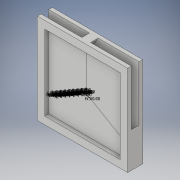
# Autodesk Inventor part: end door
Saved by Autodesk Inventor 2017 (Build 210142000, 142)
## iProperties
Created: 2018-03-09
Part Number: end door
Material: Generic
Document SubType Name: Modeling
Designer: Braxton
Density: 1 g/cm^3
Appearance: Default
Author: Braxton
Autodesk Inventor part; units mm, degrees
ref_plane "YZ Plane" through (0, 0, 0) normal (1, 0, 0) x (0, 1, 0)
ref_plane "XZ Plane" through (0, 0, 0) normal (0, 1, 0) x (-1, 0, 0)
ref_plane "XY Plane" through (0, 0, 0) normal (0, 0, 1) x (1, 0, 0)
sketch "Sketch1" plane through (0, 0, 0) normal (0, 0, 1) x (1, 0, 0)
  line L0 (0, 0) -> (2540, 0)
  line L1 (2540, 0) -> (2540, 2540)
  line L2 (2540, 2540) -> (0, 2540)
  line L3 (0, 2540) -> (0, 0)
  line L4 (-254, 2794) -> (2794, 2794)
  line L5 (2794, 2794) -> (2794, -254)
  line L6 (2794, -254) -> (-254, -254)
  line L7 (-254, -254) -> (-254, 2794)
  dimension "d0" = 2540
  dimension "d1" = 2540
  dimension "d3" = 254
  dimension "d4" = 254
  dimension "d5" = 254
  dimension "d6" = 254
  constraints: 16 end point, 4 perpendicular, 2 horizontal, 2 parallel
  measures "d0" distance of L0.start L0.end
  measures "d1" distance of L0.end L1.end
  measures "d3" distance between parallel lines of L2 L4
  measures "d4" distance between parallel lines of L3 L7
  measures "d5" distance between parallel lines of L5 L1
  measures "d6" distance between parallel lines of L6 L0
extrude "frame" add sketch "Sketch1" along normal mid plane 508
ref_plane "Work Plane3" through (0, 0, 0) normal (0, 0, 1) x (1, 0, 0)
sketch "Sketch8" plane through (0, 0, 0) normal (0, 0, 1) x (1, 0, 0)
  line L0 (2540, 0) -> (0, 0) projected
  line L1 (0, 0) -> (0, -254)
  line L2 (-254, -254) -> (2794, -254) projected
  line L3 (0, -254) -> (2540, -254)
  line L4 (2540, 2540) -> (2540, 0) projected
  line L5 (2540, -254) -> (2540, 0)
  line L6 (2540, 0) -> (0, 0)
  constraints: 8 end point, 3 perpendicular, 1 point on line, 1 vertical
extrude "door slot bottom" cut sketch "Sketch8" along normal mid plane 254
sketch "Sketch5" plane through (0, 0, 0) normal (0, 0, 1) x (1, 0, 0)
  line L0 (0, 0) -> (0, 2540) projected
  line L1 (2540, 0) -> (2540, 2540) projected
  line L2 (1270, 1143) -> (1270, 970.0002) construction
  line L3 (0, 0) -> (2540, 0) projected
  line L4 (0, 498.8101) -> (0, 0)
  line L5 (0, 0) -> (2540, 0)
  line L6 (2540, 0) -> (2540, 498.8101)
  line L7 (1270, 1232.045) -> (0, 498.8101)
  line L8 (1270, 1232.045) -> (2540, 498.8101)
  line L9 (0, 498.8101) -> (0, 2540)
  line L10 (0, 2540) -> (1270, 2540)
  line L11 (2540, 2540) -> (0, 2540) projected
  line L12 (1270, 2540) -> (1270, 1232.045)
  line L13 (1270, 2540) -> (2540, 2540)
  line L14 (2540, 2540) -> (2540, 498.8101)
  dimension "d247" = 60
  dimension "d248" = 60
  constraints: 22 end point, 3 perpendicular, 2 collinear, 2 point on line, 2 vertical, 1 horizontal, 1 midpoint
  measures "d247" angle of L7 L2
  measures "d248" angle of L8 L2
extrude "doors sketch" add sketch "Sketch5" along normal mid plane 254 separate body contours L0 L7 L8 L1 L3
extrude "top left door" add sketch "Sketch5" along normal mid plane 254 separate body contours L0 L10 L12 L7
extrude "top right door" add sketch "Sketch5" along normal mid plane 254 separate body contours L12 L11 L1 L8
sketch "Sketch7" plane through (0, 0, 0) normal (0, 0, 1) x (1, 0, 0)
  line L0 (106.265, 560.1623) -> (-264.3091, 1202.0154) construction
  line L1 (0, 498.8101) -> (-254, 938.751)
  line L2 (1270, 1232.045) -> (2540, 498.8101) projected
  line L3 (1270, 1232.045) -> (1270, 2794) construction
  line L4 (-254, 2794) -> (2794, 2794) projected
  line L5 (2540, 2540) -> (0, 2540) projected
  line L6 (1270, 2540) -> (1123.353, 2794)
  line L7 (-254, -254) -> (-254, 2794) projected
  line L8 (1123.353, 2794) -> (-254, 2794)
  line L9 (-254, 2794) -> (-254, 938.751)
  line L10 (0, 2540) -> (1270, 2540)
  line L11 (0, 498.8101) -> (1270, 1232.045) projected
  line L12 (0, 2540) -> (0, 498.8101)
  line L13 (2540, 498.8101) -> (2794, 938.751)
  line L14 (1270, 2540) -> (1416.647, 2794)
  line L15 (1416.647, 2794) -> (2794, 2794)
  line L16 (2794, 2794) -> (2794, 938.751)
  line L17 (2540, 2540) -> (1270, 2540)
  line L18 (2540, 2540) -> (2540, 498.8101)
  constraints: 28 end point, 3 point on line, 2 midpoint, 2 parallel, 2 symmetric about line, 1 horizontal, 1 perpendicular, 1 vertical
extrude "top left and right slots" cut sketch "Sketch7" along normal mid plane 254 contours L1 L7 L4 L6 L5 L12 | L18 L5 L14 L4 L16 L13 bodies 1
sketch "Sketch6" plane through (0, 0, 0) normal (0, 0, 1) x (1, 0, 0)
  line L0 (1270, 1324.5674) -> (1270, 1217.3803) construction
  line L1 (35.592, 519.3592) -> (22.892, 541.3562) construction
  line L2 (11.8934, 535.0062) -> (33.8905, 547.7062)
  line L3 (11.8934, 535.0062) -> (0, 498.8101)
  line L4 (119.4759, 538.4602) -> (106.7759, 560.4572) construction
  line L5 (108.4774, 532.1102) -> (130.4744, 544.8102)
  line L6 (71.1839, 539.9082) -> (108.4774, 532.1102)
  line L7 (33.8905, 547.7062) -> (71.1839, 539.9082)
  line L8 (130.4744, 544.8102) -> (142.3679, 581.0063)
  line L9 (1270, 1232.045) -> (2540, 498.8101) projected
  line L10 (0, 498.8101) -> (1270, 1232.045) projected
  line L11 (272.8423, 627.0063) -> (284.7357, 663.2024)
  line L12 (250.8452, 614.3063) -> (272.8423, 627.0063)
  line L13 (213.5518, 622.1043) -> (250.8452, 614.3063)
  line L14 (176.2584, 629.9023) -> (213.5518, 622.1043)
  line L15 (177.9598, 601.5553) -> (165.2598, 623.5523) construction
  line L16 (154.2613, 617.2023) -> (176.2584, 629.9023)
  line L17 (154.2613, 617.2023) -> (142.3679, 581.0063)
  line L18 (261.8438, 620.6563) -> (249.1438, 642.6534) construction
  line L19 (415.2102, 709.2024) -> (427.1036, 745.3985)
  line L20 (393.2131, 696.5024) -> (415.2102, 709.2024)
  line L21 (355.9197, 704.3004) -> (393.2131, 696.5024)
  line L22 (318.6262, 712.0985) -> (355.9197, 704.3004)
  line L23 (320.3277, 683.7514) -> (307.6277, 705.7485) construction
  line L24 (296.6292, 699.3985) -> (318.6262, 712.0985)
  line L25 (296.6292, 699.3985) -> (284.7357, 663.2024)
  line L26 (404.2116, 702.8524) -> (391.5116, 724.8495) construction
  line L27 (557.578, 791.3986) -> (569.4715, 827.5946)
  line L28 (535.581, 778.6986) -> (557.578, 791.3986)
  line L29 (498.2875, 786.4966) -> (535.581, 778.6986)
  line L30 (460.9941, 794.2946) -> (498.2875, 786.4966)
  line L31 (462.6956, 765.9475) -> (449.9956, 787.9446) construction
  line L32 (438.997, 781.5946) -> (460.9941, 794.2946)
  line L33 (438.997, 781.5946) -> (427.1036, 745.3985)
  line L34 (546.5795, 785.0486) -> (533.8795, 807.0456) construction
  line L35 (699.9459, 873.5947) -> (711.8393, 909.7908)
  line L36 (677.9488, 860.8947) -> (699.9459, 873.5947)
  line L37 (640.6554, 868.6927) -> (677.9488, 860.8947)
  line L38 (603.362, 876.4907) -> (640.6554, 868.6927)
  line L39 (605.0634, 848.1437) -> (592.3634, 870.1407) construction
  line L40 (581.3649, 863.7907) -> (603.362, 876.4907)
  line L41 (581.3649, 863.7907) -> (569.4715, 827.5946)
  line L42 (688.9474, 867.2447) -> (676.2474, 889.2417) construction
  line L43 (842.3138, 955.7908) -> (854.2072, 991.9869)
  line L44 (820.3167, 943.0908) -> (842.3138, 955.7908)
  line L45 (783.0233, 950.8888) -> (820.3167, 943.0908)
  line L46 (745.7298, 958.6868) -> (783.0233, 950.8888)
  line L47 (747.4313, 930.3398) -> (734.7313, 952.3368) construction
  line L48 (723.7328, 945.9868) -> (745.7298, 958.6868)
  line L49 (723.7328, 945.9868) -> (711.8393, 909.7908)
  line L50 (831.3152, 949.4408) -> (818.6152, 971.4379) construction
  line L51 (984.6816, 1037.9869) -> (996.5751, 1074.183)
  line L52 (962.6846, 1025.2869) -> (984.6816, 1037.9869)
  line L53 (925.3911, 1033.085) -> (962.6846, 1025.2869)
  line L54 (888.0977, 1040.883) -> (925.3911, 1033.085)
  line L55 (889.7992, 1012.5359) -> (877.0992, 1034.533) construction
  line L56 (866.1006, 1028.183) -> (888.0977, 1040.883)
  line L57 (866.1006, 1028.183) -> (854.2072, 991.9869)
  line L58 (973.6831, 1031.6369) -> (960.9831, 1053.634) construction
  line L59 (1127.0495, 1120.1831) -> (1138.9429, 1156.3791)
  line L60 (1105.0525, 1107.4831) -> (1127.0495, 1120.1831)
  line L61 (1067.759, 1115.2811) -> (1105.0525, 1107.4831)
  line L62 (1030.4656, 1123.0791) -> (1067.759, 1115.2811)
  line L63 (1032.167, 1094.732) -> (1019.467, 1116.7291) construction
  line L64 (1008.4685, 1110.3791) -> (1030.4656, 1123.0791)
  line L65 (1008.4685, 1110.3791) -> (996.5751, 1074.183)
  line L66 (1116.051, 1113.8331) -> (1103.351, 1135.8301) construction
  line L67 (1172.8334, 1205.2752) -> (1210.1269, 1197.4772)
  line L68 (1174.5349, 1176.9282) -> (1161.8349, 1198.9252) construction
  line L69 (1150.8364, 1192.5752) -> (1172.8334, 1205.2752)
  line L70 (1150.8364, 1192.5752) -> (1138.9429, 1156.3791)
  line L71 (0, 498.8101) -> (71.1839, 539.9082)
  line L72 (71.1839, 539.9082) -> (142.3679, 581.0063)
  line L73 (142.3679, 581.0063) -> (213.5518, 622.1043)
  line L74 (213.5518, 622.1043) -> (284.7357, 663.2024)
  line L75 (284.7357, 663.2024) -> (355.9197, 704.3004)
  line L76 (355.9197, 704.3004) -> (427.1036, 745.3985)
  line L77 (427.1036, 745.3985) -> (498.2875, 786.4966)
  line L78 (498.2875, 786.4966) -> (569.4715, 827.5946)
  line L79 (569.4715, 827.5946) -> (640.6554, 868.6927)
  line L80 (640.6554, 868.6927) -> (711.8393, 909.7908)
  line L81 (711.8393, 909.7908) -> (783.0233, 950.8888)
  line L82 (783.0233, 950.8888) -> (854.2072, 991.9869)
  line L83 (854.2072, 991.9869) -> (925.3911, 1033.085)
  line L84 (925.3911, 1033.085) -> (996.5751, 1074.183)
  line L85 (996.5751, 1074.183) -> (1067.759, 1115.2811)
  line L86 (1067.759, 1115.2811) -> (1138.9429, 1156.3791)
  line L87 (1138.9429, 1156.3791) -> (1210.1269, 1197.4772)
  line L88 (2409.5256, 544.8102) -> (2397.6321, 581.0063)
  line L89 (2431.5226, 532.1102) -> (2409.5256, 544.8102)
  line L90 (2468.8161, 539.9082) -> (2431.5226, 532.1102)
  line L91 (2506.1095, 547.7062) -> (2468.8161, 539.9082)
  line L92 (2504.408, 519.3592) -> (2517.108, 541.3562) construction
  line L93 (2528.1066, 535.0062) -> (2506.1095, 547.7062)
  line L94 (2528.1066, 535.0062) -> (2540, 498.8101)
  line L95 (2420.5241, 538.4602) -> (2433.2241, 560.4572) construction
  line L96 (2267.1577, 627.0063) -> (2255.2643, 663.2024)
  line L97 (2289.1548, 614.3063) -> (2267.1577, 627.0063)
  line L98 (2278.1562, 620.6563) -> (2290.8562, 642.6534) construction
  line L99 (2326.4482, 622.1043) -> (2289.1548, 614.3063)
  line L100 (2363.7416, 629.9023) -> (2326.4482, 622.1043)
  line L101 (2385.7387, 617.2023) -> (2363.7416, 629.9023)
  line L102 (2385.7387, 617.2023) -> (2397.6321, 581.0063)
  line L103 (2362.0402, 601.5553) -> (2374.7402, 623.5523) construction
  line L104 (2124.7898, 709.2024) -> (2112.8964, 745.3985)
  line L105 (2146.7869, 696.5024) -> (2124.7898, 709.2024)
  line L106 (2135.7884, 702.8524) -> (2148.4884, 724.8495) construction
  line L107 (2184.0803, 704.3004) -> (2146.7869, 696.5024)
  line L108 (2221.3738, 712.0985) -> (2184.0803, 704.3004)
  line L109 (2243.3708, 699.3985) -> (2221.3738, 712.0985)
  line L110 (2243.3708, 699.3985) -> (2255.2643, 663.2024)
  line L111 (2219.6723, 683.7514) -> (2232.3723, 705.7485) construction
  line L112 (1982.422, 791.3986) -> (1970.5285, 827.5946)
  line L113 (2004.419, 778.6986) -> (1982.422, 791.3986)
  line L114 (1993.4205, 785.0486) -> (2006.1205, 807.0456) construction
  line L115 (2041.7125, 786.4966) -> (2004.419, 778.6986)
  line L116 (2079.0059, 794.2946) -> (2041.7125, 786.4966)
  line L117 (2101.003, 781.5946) -> (2079.0059, 794.2946)
  line L118 (2101.003, 781.5946) -> (2112.8964, 745.3985)
  line L119 (2077.3044, 765.9475) -> (2090.0044, 787.9446) construction
  line L120 (1840.0541, 873.5947) -> (1828.1607, 909.7908)
  line L121 (1862.0512, 860.8947) -> (1840.0541, 873.5947)
  line L122 (1851.0526, 867.2447) -> (1863.7526, 889.2417) construction
  line L123 (1899.3446, 868.6927) -> (1862.0512, 860.8947)
  line L124 (1936.638, 876.4907) -> (1899.3446, 868.6927)
  line L125 (1958.6351, 863.7907) -> (1936.638, 876.4907)
  line L126 (1958.6351, 863.7907) -> (1970.5285, 827.5946)
  line L127 (1934.9366, 848.1437) -> (1947.6366, 870.1407) construction
  line L128 (1697.6862, 955.7908) -> (1685.7928, 991.9869)
  line L129 (1719.6833, 943.0908) -> (1697.6862, 955.7908)
  line L130 (1708.6848, 949.4408) -> (1721.3848, 971.4379) construction
  line L131 (1756.9767, 950.8888) -> (1719.6833, 943.0908)
  line L132 (1794.2702, 958.6868) -> (1756.9767, 950.8888)
  line L133 (1816.2672, 945.9868) -> (1794.2702, 958.6868)
  line L134 (1816.2672, 945.9868) -> (1828.1607, 909.7908)
  line L135 (1792.5687, 930.3398) -> (1805.2687, 952.3368) construction
  line L136 (1555.3184, 1037.9869) -> (1543.4249, 1074.183)
  line L137 (1577.3154, 1025.2869) -> (1555.3184, 1037.9869)
  line L138 (1566.3169, 1031.6369) -> (1579.0169, 1053.634) construction
  line L139 (1614.6089, 1033.085) -> (1577.3154, 1025.2869)
  line L140 (1651.9023, 1040.883) -> (1614.6089, 1033.085)
  line L141 (1673.8994, 1028.183) -> (1651.9023, 1040.883)
  line L142 (1673.8994, 1028.183) -> (1685.7928, 991.9869)
  line L143 (1650.2008, 1012.5359) -> (1662.9008, 1034.533) construction
  line L144 (1412.9505, 1120.1831) -> (1401.0571, 1156.3791)
  line L145 (1434.9475, 1107.4831) -> (1412.9505, 1120.1831)
  line L146 (1423.949, 1113.8331) -> (1436.649, 1135.8301) construction
  line L147 (1472.241, 1115.2811) -> (1434.9475, 1107.4831)
  line L148 (1509.5344, 1123.0791) -> (1472.241, 1115.2811)
  line L149 (1531.5315, 1110.3791) -> (1509.5344, 1123.0791)
  line L150 (1531.5315, 1110.3791) -> (1543.4249, 1074.183)
  line L151 (1507.833, 1094.732) -> (1520.533, 1116.7291) construction
  line L152 (1367.1666, 1205.2752) -> (1329.8731, 1197.4772)
  line L153 (1389.1636, 1192.5752) -> (1367.1666, 1205.2752)
  line L154 (1389.1636, 1192.5752) -> (1401.0571, 1156.3791)
  line L155 (1365.4651, 1176.9282) -> (1378.1651, 1198.9252) construction
  line L156 (2540, 498.8101) -> (2468.8161, 539.9082)
  line L157 (2468.8161, 539.9082) -> (2397.6321, 581.0063)
  line L158 (2397.6321, 581.0063) -> (2326.4482, 622.1043)
  line L159 (2326.4482, 622.1043) -> (2255.2643, 663.2024)
  line L160 (2255.2643, 663.2024) -> (2184.0803, 704.3004)
  line L161 (2184.0803, 704.3004) -> (2112.8964, 745.3985)
  line L162 (2112.8964, 745.3985) -> (2041.7125, 786.4966)
  line L163 (2041.7125, 786.4966) -> (1970.5285, 827.5946)
  line L164 (1970.5285, 827.5946) -> (1899.3446, 868.6927)
  line L165 (1899.3446, 868.6927) -> (1828.1607, 909.7908)
  line L166 (1828.1607, 909.7908) -> (1756.9767, 950.8888)
  line L167 (1756.9767, 950.8888) -> (1685.7928, 991.9869)
  line L168 (1685.7928, 991.9869) -> (1614.6089, 1033.085)
  line L169 (1614.6089, 1033.085) -> (1543.4249, 1074.183)
  line L170 (1543.4249, 1074.183) -> (1472.241, 1115.2811)
  line L171 (1472.241, 1115.2811) -> (1401.0571, 1156.3791)
  line L172 (1401.0571, 1156.3791) -> (1329.8731, 1197.4772)
  dimension "d326" = 25.4
  dimension "d327" = 25.4
  dimension "d328" = 38.1
  dimension "d329" = 38.1
  dimension "d330" = 38.1
  dimension "d331" = 25.4
  dimension "d332" = 38.1
  dimension "d390" = 25.4
  dimension "d391" = 25.4
  dimension "d392" = 25.4
  dimension "d393" = 38.1
  dimension "d394" = 38.1
  dimension "d395" = 38.1
  dimension "d396" = 25.4
  dimension "d397" = 38.1
  dimension "d398" = 25.4
  dimension "d399" = 25.4
  dimension "d400" = 25.4
  dimension "d401" = 38.1
  dimension "d402" = 38.1
  dimension "d403" = 38.1
  dimension "d404" = 25.4
  dimension "d405" = 38.1
  dimension "d406" = 25.4
  dimension "d407" = 25.4
  dimension "d408" = 25.4
  dimension "d409" = 38.1
  dimension "d410" = 38.1
  dimension "d411" = 38.1
  dimension "d412" = 25.4
  dimension "d413" = 38.1
  dimension "d414" = 25.4
  dimension "d415" = 25.4
  dimension "d416" = 25.4
  dimension "d417" = 38.1
  dimension "d418" = 38.1
  dimension "d419" = 38.1
  dimension "d420" = 25.4
  dimension "d421" = 38.1
  dimension "d422" = 25.4
  dimension "d423" = 25.4
  dimension "d424" = 25.4
  dimension "d425" = 38.1
  dimension "d426" = 38.1
  dimension "d427" = 38.1
  dimension "d428" = 25.4
  dimension "d429" = 38.1
  dimension "d430" = 25.4
  dimension "d431" = 25.4
  dimension "d432" = 25.4
  dimension "d433" = 38.1
  dimension "d434" = 38.1
  dimension "d435" = 38.1
  dimension "d436" = 25.4
  dimension "d437" = 38.1
  dimension "d438" = 25.4
  dimension "d439" = 25.4
  dimension "d440" = 25.4
  dimension "d441" = 38.1
  dimension "d442" = 38.1
  dimension "d443" = 38.1
  dimension "d444" = 25.4
  dimension "d445" = 38.1
  dimension "d446" = 25.4
  constraints: 344 end point, 87 symmetric about line, 18 point on line, 17 midpoint, 17 perpendicular, 1 collinear, 1 vertical, 52 other
  measures "d326" distance of L1.start L1.end
  measures "d327" distance of L2.start L7.start
  measures "d328" distance of L3.end L2.start
  measures "d329" distance of L7.start L6.start
  measures "d330" distance of L6.start L5.start
  measures "d331" distance of L5.start L8.start
  measures "d332" distance of L8.start L8.end
  measures "d390" distance of L4.start L4.end
  measures "d391" distance of L15.start L15.end
  measures "d392" distance of L16.start L14.start
  measures "d393" distance of L8.end L16.start
  measures "d394" distance of L14.start L13.start
  measures "d395" distance of L13.start L12.start
  measures "d396" distance of L12.start L11.start
  measures "d397" distance of L11.start L11.end
  measures "d398" distance of L18.start L18.end
  measures "d399" distance of L23.start L23.end
  measures "d400" distance of L24.start L22.start
  measures "d401" distance of L11.end L24.start
  measures "d402" distance of L22.start L21.start
  measures "d403" distance of L21.start L20.start
  measures "d404" distance of L20.start L19.start
  measures "d405" distance of L19.start L19.end
  measures "d406" distance of L26.start L26.end
  measures "d407" distance of L31.start L31.end
  measures "d408" distance of L32.start L30.start
  measures "d409" distance of L19.end L32.start
  measures "d410" distance of L30.start L29.start
  measures "d411" distance of L29.start L28.start
  measures "d412" distance of L28.start L27.start
  measures "d413" distance of L27.start L27.end
  measures "d414" distance of L34.start L34.end
  measures "d415" distance of L39.start L39.end
  measures "d416" distance of L40.start L38.start
  measures "d417" distance of L27.end L40.start
  measures "d418" distance of L38.start L37.start
  measures "d419" distance of L37.start L36.start
  measures "d420" distance of L36.start L35.start
  measures "d421" distance of L35.start L35.end
  measures "d422" distance of L42.start L42.end
  measures "d423" distance of L47.start L47.end
  measures "d424" distance of L48.start L46.start
  measures "d425" distance of L35.end L48.start
  measures "d426" distance of L46.start L45.start
  measures "d427" distance of L45.start L44.start
  measures "d428" distance of L44.start L43.start
  measures "d429" distance of L43.start L43.end
  measures "d430" distance of L50.start L50.end
  measures "d431" distance of L55.start L55.end
  measures "d432" distance of L56.start L54.start
  measures "d433" distance of L43.end L56.start
  measures "d434" distance of L54.start L53.start
  measures "d435" distance of L53.start L52.start
  measures "d436" distance of L52.start L51.start
  measures "d437" distance of L51.end L51.start
  measures "d438" distance of L58.start L58.end
  measures "d439" distance of L63.start L63.end
  measures "d440" distance of L64.start L62.start
  measures "d441" distance of L51.end L64.start
  measures "d442" distance of L62.start L61.start
  measures "d443" distance of L61.start L60.start
  measures "d444" distance of L60.start L59.start
  measures "d445" distance of L59.start L59.end
  measures "d446" distance of L66.start L66.end
equation "\"d3\" = d4"
equation "\"d5\" = d4"
equation "\"d6\" = d4"
